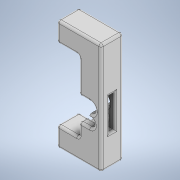
# Autodesk Inventor part: Slider
Saved by Autodesk Inventor 2022 (Build 260153000, 153)
## iProperties
Created: 2022-03-29
Part Number: Slider
Material: Generic
Document SubType Name: Modeling
Designer: thoms
Density: 1 g/cm^3
Appearance: Default
Author: thoms
Autodesk Inventor part; units mm, degrees
ref_plane "YZ Plane" through (0, 0, 0) normal (1, 0, 0) x (0, 1, 0)
ref_plane "XZ Plane" through (0, 0, 0) normal (0, 1, 0) x (-1, 0, 0)
ref_plane "XY Plane" through (0, 0, 0) normal (0, 0, 1) x (1, 0, 0)
sketch "Sketch1" plane through (0, 0, 0) normal (0, 0, 1) x (1, 0, 0)
  line L0 (-25, 12.5) -> (-15, 12.5)
  line L1 (-15, 12.5) -> (-15, -12.5)
  line L2 (-15, -12.5) -> (-25, -12.5)
  line L3 (-25, -12.5) -> (-25, 12.5)
  line L4 (-25, 8) -> (-20, 8)
  line L5 (-20, 8) -> (-20, -8)
  line L6 (-20, -8) -> (-25, -8)
  line L7 (-25, -8) -> (-25, 8)
  point P0 (0, 0)
  dimension "d0" = 25
  dimension "d1" = 12.5
  dimension "d3" = 25
  dimension "d4" = 5
  dimension "d5" = 16
  dimension "d6" = 8
  dimension "d7" = 0
  dimension "d21" = 5
  constraints: 16 end point, 4 parallel, 2 horizontal, 2 perpendicular
  measures "d0" distance of L0.end L1.end
  measures "d1" distance from line of point (0, 0) L0
  measures "d3" distance from line of point (0, 0) L3
  measures "d4" distance between parallel lines of L1 L5
  measures "d5" distance of L4.end L5.end
  measures "d6" distance from line of point (0, 0) L4
  measures "d7" distance between parallel lines of L3 L7
  measures "d21" distance between parallel lines of L5 L3
extrude "Extrusion1" add sketch "Sketch1" against normal blind 5 contours L0 L1 L2 L3 L6 L5 L4
fillet "Fillet1" radius 0.5 24 edges at (-22.5, -8, 0) (-20, 0, 0) (-22.5, 8, 0) (-15, 0, 0) (-15, 0, -5) (-20, 0, -5) (-15, 12.5, -2.5) (-15, -12.5, -2.5) (-20, -12.5, 0) (-20, -8, -2.5) (-20, 8, -2.5) (-20, -12.5, -5) (-22.5, -8, -5) (-20, 12.5, 0) (-20, 12.5, -5) (-25, -10.25, 0) (-25, -12.5, -2.5) (-25, -10.25, -5) (-25, -8, -2.5) (-25, 8, -2.5) (-25, 10.25, 0) (-25, 12.5, -2.5) (-25, 10.25, -5) (-22.5, 8, -5)
sketch "Sketch2" plane through (-15, -12, -0.5) normal (1, 0, 0) x (0, 0, -1)
  line L0 (1.425, 13.6) -> (2.575, 13.6)
  line L1 (2.575, 13.6) -> (2.575, 6.35)
  line L2 (2.575, 6.35) -> (1.425, 6.35)
  line L3 (1.425, 6.35) -> (1.425, 13.6)
  line L4 (0.8293, 6) -> (3.4454, 6)
  line L5 (0.8293, 18) -> (3.4454, 18)
  line L6 (0, 20) -> (4, 20) projected
  line L7 (4.5, 0) -> (4.5, 24) projected
  point P0 (-0.5, 12)
  dimension "d11" = 7.25
  dimension "d12" = 1.15
  dimension "d14" = 12
  dimension "d15" = 2
  dimension "d16" = 7.6
  dimension "d17" = 1.925
  constraints: 12 end point, 3 horizontal, 2 parallel, 1 perpendicular
  measures "d11" distance of L0.end L1.end
  measures "d12" distance of L0.start L0.end
  measures "d14" distance between parallel lines of L4 L5
  measures "d15" distance between parallel lines of L6 L5
  measures "d16" distance between parallel lines of L4 L0
  measures "d17" distance between parallel lines of L7 L1
extrude "Extrusion2" cut sketch "Sketch2" against normal up to surface (5 mm away)
sketch "Sketch3" plane through (0, 0, 0) normal (0, 0, 1) x (1, 0, 0)
  arc A0 (-17.5859, -2.25) -> (-17.5859, 0.25) centre (-17.5859, -1) ccw
  arc A1 (-17.5859, -4.9) -> (-17.5859, -2.9) centre (-17.5859, -3.9) ccw
  line L0 (-21.0491, -5.65) -> (-14.6152, -5.65) construction
  line L1 (-21.0491, 1.6) -> (-14.3074, 1.6) construction
  line L2 (-17.5859, 0.25) -> (-20, 0.25)
  line L3 (-20, -7.5) -> (-20, 7.5) projected
  line L4 (-17.5859, -2.25) -> (-17.5859, -2.9)
  line L5 (-17.5859, -4.9) -> (-20, -4.9)
  line L6 (-20, 0.25) -> (-20, -4.9)
  point P0 (0, 0)
  dimension "d25" = 2
  dimension "d26" = 2.5
  dimension "d28" = 2.9
  dimension "d29" = 2.6
  constraints: 12 end point, 4 point on circle, 2 centre point, 2 horizontal, 2 perpendicular, 2 point on line, 1 parallel, 1 tangent
  measures "d25" diameter of A1
  measures "d26" diameter of A0
  measures "d28" distance of A0.centre A1.centre
  measures "d29" distance from line of L1 A0.centre
extrude "Extrusion3" cut sketch "Sketch3" against normal up to surface (5 mm away)
fillet "Fillet2" radius 0.5 34 edges at (-20, -5.275, -1.925) (-20, 0.925, -1.925) (-20, 1.6, -2.5) (-20, -5.275, -3.075) (-20, 0.925, -3.075) (-20, -5.65, -2.5) (-15, -2.025, -1.925) (-15, 1.6, -2.5) (-15, -2.025, -3.075) (-15, -5.65, -2.5) (-18.5429, 0.25, -5) (-19.8536, 0.25, -4.8536) (-20, 0.25, -3.7875) (-16.3359, -1, -5) (-18.7929, 0.25, -3.075) (-16.3359, -1, -3.075) (-18.7929, 0.25, -1.925) (-16.3359, -1, -1.925) (-18.5429, 0.25, 0) (-19.8536, 0.25, -0.1464) (-20, 0.25, -1.2125) (-16.3359, -1, 0) (-18.5429, -4.9, -5) (-19.8536, -4.9, -4.8536) (-20, -4.9, -3.7875) (-16.5859, -3.9, -5) (-18.7929, -4.9, -3.075) (-16.5859, -3.9, -3.075) (-18.7929, -4.9, -1.925) (-16.5859, -3.9, -1.925) (-18.5429, -4.9, 0) (-19.8536, -4.9, -0.1464) (-20, -4.9, -1.2125) (-16.5859, -3.9, 0)
body "Solid1"
